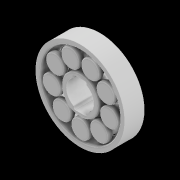
# Autodesk Inventor part: PIP-KL_parametriserad_02
Saved by Autodesk Inventor 2020 (Build 240168000, 168)
## iProperties
Created: 2020-11-21
Part Number: PIP-KL_parametriserad_02
Material: Generic
Document SubType Name: Modeling
Designer: Gottfrid
Density: 1 g/cm^3
Appearance: Default
d_inreRing: 2.500 mm
d_yttreRing: 2.500 mm
r_yttre: 10.000 mm
h_rullager: 5.000 mm
Author: Gottfrid
Autodesk Inventor part; units mm, degrees
ref_plane "YZ Plane" through (0, 0, 0) normal (1, 0, 0) x (0, 1, 0)
ref_plane "XZ Plane" through (0, 0, 0) normal (0, 1, 0) x (-1, 0, 0)
ref_plane "XY Plane" through (0, 0, 0) normal (0, 0, 1) x (1, 0, 0)
sketch "Sketch1" plane through (0, 0, 0) normal (0, 0, 1) x (1, 0, 0)
  circle A0 centre (0, 0) radius 3.5
  circle A1 centre (0, 0) radius 4.75
  circle A2 centre (0, 0) radius 10
  circle A3 centre (0, 0) radius 11.25
  circle A4 centre (0, -7.375) radius 2.375
  line L0 (1.2333, -3.7857) -> (-1.2333, -3.7857)
  line L1 (-1.6333, -3.3857) -> (-1.6333, 3.3857)
  line L2 (-1.2333, 3.7857) -> (1.2333, 3.7857)
  line L3 (1.6333, 3.3857) -> (1.6333, -3.3857)
  line L4 (1.6333, -3.7857) -> (-1.6333, 3.7857) construction
  line L5 (-1.6333, -3.7857) -> (1.6333, 3.7857) construction
  arc A5 (-1.2333, 3.7857) -> (-1.6333, 3.3857) centre (-1.2333, 3.3857) ccw
  arc A6 (1.6333, 3.3857) -> (1.2333, 3.7857) centre (1.2333, 3.3857) ccw
  arc A7 (1.2333, -3.7857) -> (1.6333, -3.3857) centre (1.2333, -3.3857) ccw
  arc A8 (-1.6333, -3.3857) -> (-1.2333, -3.7857) centre (-1.2333, -3.3857) ccw
  point P0 (-1.6333, 3.0955)
  point P1 (1.6333, 3.0955)
  point P2 (1.6333, -3.0955)
  point P3 (-1.6333, -3.0955)
  dimension "d0" = 7
  dimension "d1" = 9.5
  dimension "d2" = 20
  dimension "d3" = 22.5
  dimension "d4" = 7.375
  dimension "d5" = 4.75
  dimension "d64" = 7.5714
  dimension "d65" = 3.2667
  dimension "d66" = 0.4
  constraints: 12 end point, 9 centre point, 8 point on circle, 8 point on line, 8 tangent, 4 coincident, 3 equal radius, 2 midpoint, 2 parallel, 1 horizontal, 1 perpendicular, 1 vertical alignment
  measures "d0" diameter of A0
  measures "d1" diameter of A1
  measures "d2" diameter of A2
  measures "d3" diameter of A3
  measures "d4" distance of A4.centre point (0, 0)
  measures "d5" diameter of A4
  measures "d64" distance between parallel lines of L0 L2
  measures "d65" distance between parallel lines of L3 L1
  measures "d66" radius of A5
extrude "Extrusion1" add sketch "Sketch1" along normal blind 1 contours A0 L3 | L3 A0 L1 | A0 L1 A5 L2 A6 L3 | L3 A7 L0 A8 L1 A0 | L1 A0 | A1
extrude "Extrusion8" add sketch "Sketch1" along normal blind 1 contours A4
extrude "Extrusion9" add sketch "Sketch1" along normal blind 1 contours A3
sketch "Sketch17" plane through (0, 0, 1) normal (0, 0, 1) x (1, 0, 0)
  circle A0 centre (0, 0) radius 4.75 projected
extrude "Extrusion10" add sketch "Sketch17" along normal blind 1 draft 35
sketch "Sketch18" plane through (0, -7.375, 1) normal (0, 0, 1) x (1, 0, 0)
  circle A0 centre (0, 0) radius 2.375 projected
  point P0 (0, 7.375)
extrude "Extrusion11" add sketch "Sketch18" along normal blind 1 draft -35
sketch "Sketch19" plane through (0, 0, 1) normal (0, 0, 1) x (1, 0, 0)
  circle A0 centre (0, 0) radius 10 projected
  circle A1 centre (0, 0) radius 11.25 projected
extrude "Extrusion12" add sketch "Sketch19" along normal blind 1 draft 35
sketch "Sketch20" plane through (0, 0, 2) normal (0, 0, 1) x (1, 0, 0)
  circle A0 centre (0, 0) radius 5.4502 projected
extrude "Extrusion13" add sketch "Sketch20" along normal blind 0.5
sketch "Sketch21" plane through (0, -7.375, 2) normal (0, 0, 1) x (1, 0, 0)
  circle A0 centre (0, 0) radius 1.6748 projected
  point P0 (0, 7.375)
extrude "Extrusion14" add sketch "Sketch21" along normal blind 0.5
sketch "Sketch22" plane through (0, 0, 2) normal (0, 0, 1) x (1, 0, 0)
  circle A0 centre (0, 0) radius 9.2998 projected
  circle A1 centre (0, 0) radius 11.9502 projected
extrude "Extrusion15" add sketch "Sketch22" along normal blind 0.5
chamfer "Chamfer6" distance 0.2 angle 45 1 edges at (-10, 0, 0)
chamfer "Chamfer2" distance 0.2 angle 45 1 edges at (-2.375, -7.375, 0)
chamfer "Chamfer5" distance 0.2 angle 45 1 edges at (-4.75, 0, 0)
mirror "Mirror1" about plane through (0, 0, 2.5) normal (0, 0, 1) of "Extrusion13", "Extrusion10", "Extrusion1", "Chamfer5"
mirror "Mirror2" about plane through (0, -7.375, 2.5) normal (0, 0, 1) of "Extrusion8", "Extrusion11", "Extrusion14", "Chamfer2"
mirror "Mirror3" about plane through (0, 0, 2.5) normal (0, 0, 1) of "Extrusion9", "Extrusion12", "Extrusion15", "Chamfer6"
extrude "Extrusion18" cut sketch "Sketch1" along normal blind 999 contours A0 L1 A5 L2 A6 L3 | L3 A7 L0 A8 L1 A0
pattern_circular "Circular Pattern3" count 9 over 360 about axis through (0, 0, -10) along (0, 0, 1) of "Extrusion8", "Extrusion11", "Extrusion14", "Chamfer2", "Mirror2"
extrude "Extrusion19" cut sketch "Sketch1" along normal blind 999 contours A0 L3 | L3 A0 L1 | L1 A0
extrude "Extrusion20" cut sketch "Sketch1" along normal blind 999 contours A0 L3 | L3 A0 L1 | A0 L1 A5 L2 A6 L3 | L3 A7 L0 A8 L1 A0 | L1 A0 | A1 | A2 | A3 | A4 keep common part
equation "\"d0\" = D_axel"
equation "\"d1\" = D_axel + d_inreRing"
equation "\"d2\" = 2 * r_yttre"
equation "\"d3\" = 2 * r_yttre + d_yttreRing"
equation "\"d4\" = beräknad_avstånd_origo_till_rullkopp"
equation "\"d5\" = beräknad_diameter_rullkropp"
equation "\"d66\" = r_filletAxel"
equation "\"d6\" = extrude_h1"
equation "\"d29\" = extrude_h1"
equation "\"d31\" = extrude_h1"
equation "\"d33\" = extrude_h1"
equation "\"d34\" = extrude_angle35"
equation "\"d35\" = extrude_h1"
equation "\"d36\" = -extrude_angle35"
equation "\"d37\" = extrude_h1"
equation "\"d38\" = extrude_angle35"
equation "\"d39\" = 0.5 * extrude_h1"
equation "\"d41\" = 0.5 * extrude_h1"
equation "\"d43\" = 0.5 * extrude_h1"
equation "\"d72\" = 0.2 * extrude_h1"
equation "\"d45\" = 0.2 * extrude_h1"
equation "\"d69\" = 0.2 * extrude_h1"
equation "\"r_inre\" = 0.5 * D_axel"
equation "\"d_inreRing\" = 2.5"
equation "\"r_yttre\" = 10"
equation "\"d_yttreRing\" = 2.5"
equation "\"d_toleransMellanRullkroppOchRing\" = 0.25"
equation "\"extrude_h1\" = 0.2 * h_rullager"
equation "\"extrude_angle35\" = 35deg"
equation "\"beräknad_diameter_rullkropp\" = r_yttre - 0.5 * d_inreRing - r_inre - 2 * d_toleransMellanRullkroppOchRing"
equation "\"beräknad_avstånd_origo_till_rullkopp\" = 0.5 * d_inreRing + r_inre + 0.5 * beräknad_diameter_rullkropp + d_toleransMellanRullkroppOchRing"
equation "\"h_rullager\" = 5"
equation "\"D_axel\" = 7"
equation "\"r_filletAxel\" = 0.4"
body "Solid1"
